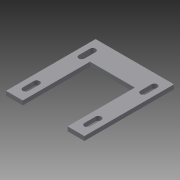
# Autodesk Inventor part: torchMount_back
Saved by Autodesk Inventor 2013 (Build 170138000, 138)
## iProperties
Created: 2012-12-09
Part Number: torchMount_back
Material: Generic
Document SubType Name: Modeling
Designer: Istvan
Density: 1 g/cm^3
Author: Istvan
Autodesk Inventor part; units mm, degrees
ref_plane "YZ Plane" through (0, 0, 0) normal (1, 0, 0) x (0, 1, 0)
ref_plane "XZ Plane" through (0, 0, 0) normal (0, 1, 0) x (-1, 0, 0)
ref_plane "XY Plane" through (0, 0, 0) normal (0, 0, 1) x (1, 0, 0)
sketch "Sketch1" plane through (0, 0, 0) normal (0, 1, 0) x (-1, 0, 0)
  line L0 (0, 0) -> (44.45, 0)
  line L1 (0, 101.6) -> (0, 0)
  line L2 (44.45, 25.4) -> (19.05, 25.4)
  line L3 (19.05, 25.4) -> (19.05, 101.6)
  line L4 (44.45, 25.4) -> (44.45, 0)
  line L5 (19.05, 101.6) -> (0, 101.6)
  line L6 (12.827, 88.9) -> (12.827, 76.2)
  line L7 (6.223, 76.2) -> (6.223, 88.9)
  arc A0 (12.827, 88.9) -> (6.223, 88.9) centre (9.525, 88.9) ccw
  arc A1 (6.223, 76.2) -> (12.827, 76.2) centre (9.525, 76.2) ccw
  line L8 (12.827, 25.4) -> (12.827, 12.7)
  line L9 (6.223, 12.7) -> (6.223, 25.4)
  arc A2 (12.827, 25.4) -> (6.223, 25.4) centre (9.525, 25.4) ccw
  arc A3 (6.223, 12.7) -> (12.827, 12.7) centre (9.525, 12.7) ccw
  dimension "d1" = 101.6
  dimension "d3" = 19.05
  dimension "d8" = 44.45
  dimension "d9" = 25.4
  dimension "d11" = 6.604
  dimension "d12" = 6.223
  dimension "d13" = 6.223
  dimension "d14" = 12.7
  dimension "d15" = 12.7
  dimension "d16" = 6.604
  dimension "d17" = 12.7
  dimension "d18" = 12.7
  constraints: 20 end point, 8 point on circle, 8 tangent, 4 centre point, 3 parallel, 2 vertical, 1 horizontal, 1 vertical alignment
  measures "d1" distance of L1.start L0.start
  measures "d3" distance between parallel lines of L1 L3
  measures "d8" distance between parallel lines of L4 L1
  measures "d9" distance between parallel lines of L0 L2
  measures "d11" distance between parallel lines of L6 L7
  measures "d12" distance between parallel lines of L1 L7
  measures "d13" distance between parallel lines of L3 L6
  measures "d14" distance of A1.centre A0.centre
  measures "d15" distance from line of L5 A0.centre
  measures "d16" distance between parallel lines of L8 L9
  measures "d17" distance of A3.centre A2.centre
  measures "d18" distance from line of L0 A3.centre
extrude "Extrusion1" add sketch "Sketch1" against normal blind 4.7625
mirror "Mirror1" about plane through (-44.45, 0, 25.4) normal (-1, 0, 0)
equation "\"d3\" = d4"
equation "\"d12\" = d13"
equation "\"d4\" = 19.05"
body "Solid1"
